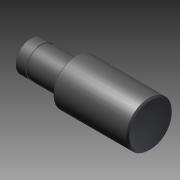
# Autodesk Inventor part: SFRX15-25-F15-B5-P10
Saved by Autodesk Inventor 2011 SP1 (Build 150282100, 282)
## iProperties
Created: 2016-06-25
Part Number: SFRX15-25-F15-B5-P10
Catalog Web Link: www.cadenas.de
Description: SFRX, PSFRX, SSFRX-Rotary Shafts - One End Stepped with Retaining Ring Groove -
Vendor: MISUMI
Document SubType Name: Modeling
Designer: psAdmin
Manufacturer: MISUMI
Mass: 5.57384 g
Surface Area: 19.7317 cm^2
Volume: 5.57384 cm^3
Density: 1 g/cm^3
Category: PARTsolutions
Company: MISUMI
Title: SFRX15-25-F15-B5-P10
Author: Cadenas PARTsolutions
Comments: Rotary Shafts - One End Stepped with Retaining Ring Groove -
PSOL_IDENT_0: {$CADENAS_DATA\23d-libs\misumi\metric\11_rotary_shafts\sfrx.prj},280 {VTYP=3D},{NB=SFRX15-25-F15-B5-
PSOL_IDENT_1: P10},{LINA=SFRX15-25-F15-B5-P10},{NN=SFRX, PSFRX, SSFRX},{DATE=27.05.2016 14:10:13},{GEOMDATE=20.01.
PSOL_IDENT_2: 2016 00:25:22},{VERSION=},{LINEID=70},{LINESUBID=-1},{WBVAR=MAT,ST,ALT1,L,F,B,P,ALT2,KC,A,WKC,C,K,E,
PSOL_IDENT_3: ALT3,FC,GALT3,WFC,J,W,V,ALT4,SFC,SG,AG,ALT5,UC}  {NB=SFRX15-25-F15-B5-P10},{LINA=SFRX15-25-F15-B5-P1
PSOL_IDENT_4: 0},{KT=DUMMY},{PN=SFRX15-25-F15-B5-P10},{TYPE=SFRX},{MAT=S45C},{MATALG= 'S45C','S45C Equivalent', 'S
PSOL_IDENT_5: US304','SUS304' },{ST=BO},{STALG= 'BO','Black Oxide', 'ENP','Electroless Nickel Plating' },{D=15},{A
PSOL_IDENT_6: LT1=},{L=25.0},{LALG=[25:696/0.1]},{LMIN=25},{LMAX=696},{F=15.0},{FALG=[4:70/0.1]},{FMIN=4},{FMAX=70
PSOL_IDENT_7: },{B=5},{BMAX=13},{BMIN=2},{BALG=[2:13/1]},{P=10},{PALG=[5:14/1]},{PMAX=14},{PMAX1=14},{PMIN=5},{PMI
PSOL_IDENT_8: N1=3},{CIFC=0},{MM=1.15},{DD=9.6},{Y=800},{CC=0.5},{ALT2=},{ALT2ALG= '', 'w/o Key Grooves','KC','wit
PSOL_IDENT_9: h KC (Key Groove)','WKC','with WKC (Two Key Grooves)','KCWKC','with KC + WKC (Three Key Grooves)' },
PSOL_IDENT_10: {ALT2PN=},{KC=0.0},{KCALG=[0]},{KCMIN=0},{KCMAX1=20},{KCMAX2=10},{KCMAX3=5},{A=0.0},{AALG=[0]},{AMIN=
PSOL_IDENT_11: 5},{AMAX1=25},{AMAX2=15},{AMAX3=10},{WKC=0.0},{WKCALG=[0]},{WKCMIN1=0},{WKCMIN2=0},{WKCMAX1=15},{WKC
PSOL_IDENT_12: MAX2=10},{C=0.0},{CALG=[0]},{CMIN=5},{CMAX1=20},{CMAX2=15},{K=0.0},{KALG=[0]},{KMIN1=0},{KMIN2=5},{K
PSOL_IDENT_13: MAX1=20},{E=0.0},{EALG=[0]},{EMIN=5},{EMAX=25},{BB=5},{TT=3},{CIFR=0},{CIFKC=0},{CIFWKC=0},{CIFK=0},
PSOL_IDENT_14: {CIKC=0},{ALT3=},{ALT3ALG= '', 'w/o Set Screw Flat','FC','with FC (Adds a Set Screw Flat)','WFC','wi
PSOL_IDENT_15: th WFC (Adds Two Set Screw Flats)','FCWFC','with FC + WFC (Adds Three Set Screw Flats)' },{ALT3PN=},
PSOL_IDENT_16: {FC=0},{FCALG=[0]},{FCMIN=0},{FCMAX=24},{GALT3=0},{GALT3ALG=[0]},{GALT3MIN=1},{GALT3MAX=25},{GALT3MA
PSOL_IDENT_17: X2=19},{GALT3MAX3=22},{WFC=0},{WFCALG=[0]},{WFCMIN=0},{WFCMIN2=2},{WFCMAX=21},{WFCMAX2=-3},{WFCMAX3=
PSOL_IDENT_18: -4},{J=0},{JALG=[0]},{JMIN=1},{JMAX=22},{JMAX2=-2},{JMAX3=-5},{W=0},{WALG=[0]},{WMIN=0},{WMIN2=27},{
PSOL_IDENT_19: WMAX=22},{WMAX2=22},{V=0},{VALG=[0]},{VMIN=1},{VMAX=23},{VMAX2=23},{CIFCUT=0},{CIFFC=0},{ALT4=},{ALT
PSOL_IDENT_20: 4ALG= '', 'w/o SFC (2 Set Screw Flats (Angle Specified))', 'SFC' , 'with SFC (2 Set Screw Flats (Ang
PSOL_IDENT_21: le Specified))'},{ALT4PN=},{SFC=0},{SFCALG=[0]},{SFCMIN=0},{SFCMAX=24},{SG=0},{SGALG=[0]},{SGMIN=1},
PSOL_IDENT_22: {SGMAX=25},{AG=0},{AGALG=[0]},{H=0},{CIFSFC=0},{ALT5=},{ALT5ALG= '','Not applicable' },{ALT5PN=},{UC=
PSOL_IDENT_23: 0},{UCALG=[0]},{UCMIN=1},{UCMAX=19},{DDALT5=0},{LL1=0},{ERRORPN=},{ERRORALT2=OK},{ERRORALT23=OK},{ER
PSOL_IDENT_24: RORALT24=OK},{ERRORALT25=OK},{ERRORALT35=OK},{ERRORALT34=OK},{ERRORALT45=OK},{CIFKG=0},{KGMIN1=0},{K
PSOL_IDENT_25: GMAX1=0},{KGMIN2=0},{KGMAX2=0},{KGMIN3=0},{KGMAX3=0},{CIFKGC=0},{CIFKG1=1},{CIFKG2=0},{CIFKG3=0},{CI
PSOL_IDENT_26: FCALC1=0},{CIFCALC2=0},{CIFCALC3=0},{CIFKGPCUT=0},{PCUT3D=0}
NN: SFRX, PSFRX, SSFRX
NT: Rotary Shafts - One End Stepped with Retaining Ring Groove -
NB: SFRX15-25-F15-B5-P10
NBSYN: $PN.
LINA: SFRX15-25-F15-B5-P10
PN: SFRX15-25-F15-B5-P10
MAT: S45C Equivalent
ST: Black Oxide
D: 15
ALT1: w/o LKC (Changes L Tolerance)
L: 25.0
F: 15.0
B: 5
P: 10
Y: 800
ALT2: w/o Key Grooves
KC: 0.0
A: 0.0
WKC: 0.0
C: 0.0
K: 0.0
E: 0.0
ALT3: w/o Set Screw Flat
FC: 0
GALT3: 0
WFC: 0
J: 0
W: 0
V: 0
ALT4: w/o SFC (2 Set Screw Flats (Angle Specified))
SFC: 0
SG: 0
AG: 0
H: 0
ALT5: Not applicable
UC: 0
DDALT5: 0
LL1: 0
SUPPLIER: MISUMI
ARTICLENO: SFRX15-25-F15-B5-P10
BOMINFO: SFRX15-25-F15-B5-P10
CREATOR: CADENAS GmbH
Autodesk Inventor part; units mm, degrees
ref_plane "YZ Plane" through (0, 0, 0) normal (1, 0, 0) x (0, 1, 0)
ref_plane "XZ Plane" through (0, 0, 0) normal (0, 1, 0) x (-1, 0, 0)
ref_plane "XY Plane" through (0, 0, 0) normal (0, 0, 1) x (1, 0, 0)
sketch "Sketch_1" plane through (0, 0, 0) normal (0, 0, 1) x (1, 0, 0)
  line L0 (25, 0) -> (-15, 0)
  line L1 (-15, 0) -> (-15, 4.5)
  line L2 (-15, 4.5) -> (-14.5, 5)
  line L3 (-14.5, 5) -> (-0.2, 5)
  arc A0 (-0.2, 5) -> (0, 5.2) centre (-0.2, 5.2) ccw
  line L4 (0, 5.2) -> (0, 7)
  line L5 (0, 7) -> (0.5, 7.5)
  line L6 (0.5, 7.5) -> (24.5, 7.5)
  line L7 (24.5, 7.5) -> (25, 7)
  line L8 (25, 7) -> (25, 0)
  line L9 (25, 0) -> (-15, 0)
  constraints: 20 end point, 2 point on circle, 1 centre point
revolve "Revolution1" add sketch "Sketch_1" angle 360 about axis through (25, 0, 0) along (1, 0, 0)
sketch "Sketch_40" plane through (0, 0, 0) normal (0, 0, 1) x (1, 0, 0)
  line L0 (1000, 0) -> (-1000, 0)
  line L1 (-11.15, 4.8) -> (-10, 4.8)
  line L2 (-10, 4.8) -> (-10, 20)
  line L3 (-10, 20) -> (-11.15, 20)
  line L4 (-11.15, 20) -> (-11.15, 4.8)
  constraints: 10 end point
revolve "Revolution2" cut sketch "Sketch_40" angle 360 about axis through (1000, 0, 0) along (1, 0, 0)
body "Solid1"
